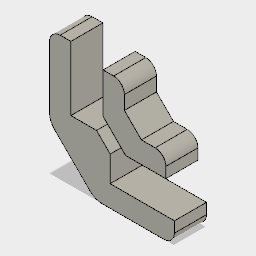
Corner Connector v15 (Autodesk Fusion 360 design; units mm, degrees)
Autodesk Fusion 360 part; units mm, degrees
sketch "Sketch1" plane through (0, 0, 0) normal (0, 0, 1) x (1, 0, 0) in component "InsideClamp"
  line L0 (0, 0) -> (23.8125, 0)
  line L1 (23.8125, 0) -> (37.2829, -13.4704)
  line L2 (37.2829, -13.4704) -> (37.2829, -37.2829)
  line L3 (37.2829, -37.2829) -> (30.9329, -37.2829)
  line L4 (0, 0) -> (0, -6.35)
  line L5 (6.35, -12.7) -> (14.4801, -12.7)
  line L6 (14.4801, -12.7) -> (24.5829, -22.8028)
  line L7 (24.5829, -22.8028) -> (24.5829, -30.9329)
  arc A0 (0, -6.35) -> (6.35, -12.7) centre (6.35, -6.35) ccw
  arc A1 (24.5829, -30.9329) -> (30.9329, -37.2829) centre (30.9329, -30.9329) ccw
  point P0 (24.5829, -37.2829)
  point P1 (0, -12.7)
  dimension "d19" = 23.8125
  dimension "d20" = 19.05
  dimension "d21" = 23.8125
  dimension "d22" = 135
  dimension "d23" = 135
  dimension "d24" = 12.7
  dimension "d25" = 12.7
  dimension "d26" = 135
  dimension "d27" = 135
  dimension "d28" = 14.2875
  dimension "d29" = 6.35
  dimension "d30" = 6.35
  measures "d19" distance of L0.start L0.end
  measures "d20" distance of L0.end L1.end
  measures "d21" distance of L1.end L2.end
  measures "d22" angle of L0 L1
  measures "d23" angle of L1 L2
  measures "d24" distance of L2.end P0
  measures "d25" distance of L0.start P1
  measures "d26" angle of L5 L6
  measures "d27" angle of L6 L7
  measures "d28" distance of L5.end L6.end
  measures "d29" radius of A0
  measures "d30" radius of A1
sketch "Sketch1 (2)" plane through (0, 0, 0) normal (0, 0, 1) x (1, 0, 0) in component "OutsideClamp"
  line L0 (-5.0893, 19.05) -> (33.0107, 19.05)
  line L1 (33.0107, 3.81) -> (41.0929, -4.2722)
  line L2 (56.3329, -4.2722) -> (56.3329, -42.3722)
  line L3 (56.3329, -42.3722) -> (62.6829, -42.3722)
  line L4 (69.0329, -36.0222) -> (69.0329, 0.6008)
  line L5 (66.0571, 7.785) -> (45.0679, 28.7742)
  line L6 (37.8837, 31.75) -> (1.2607, 31.75)
  line L7 (-5.0893, 25.4) -> (-5.0893, 19.05)
  arc A0 (1.2607, 31.75) -> (-5.0893, 25.4) centre (1.2607, 25.4) ccw
  arc A1 (62.6829, -42.3722) -> (69.0329, -36.0222) centre (62.6829, -36.0222) ccw
  line L8 (0, 0) -> (23.8125, 0)
  line L9 (37.2829, -13.4704) -> (37.2829, -37.2829)
  line L10 (33.0107, 19.05) -> (33.0107, 3.81)
  line L11 (56.3329, -4.2722) -> (41.0929, -4.2722)
  arc A2 (45.0679, 28.7742) -> (37.8837, 31.75) centre (37.8837, 21.59) ccw
  arc A3 (69.0329, 0.6008) -> (66.0571, 7.785) centre (58.8729, 0.6008) ccw
  point P0 (69.0329, -42.3722)
  point P1 (69.0329, 4.8092)
  point P2 (42.0921, 31.75)
  point P3 (-5.0893, 31.75)
  dimension "d32" = 38.1
  dimension "d38" = 135
  dimension "d39" = 135
  dimension "d42" = 6.35
  dimension "d43" = 6.35
  dimension "d44" = 12.7
  dimension "d46" = 12.7
  dimension "d47" = 38.1
  dimension "d49" = 19.05
  dimension "d50" = 19.05
  dimension "d51" = 15.24
  dimension "d52" = 15.24
  dimension "d53" = 135
  dimension "d54" = 38.1
  dimension "d55" = 11.43
  dimension "d56" = 10.16
  measures "d32" distance of L0.start L0.end
  measures "d38" angle of L4 L5
  measures "d39" angle of L5 L6
  measures "d42" radius of A0
  measures "d43" radius of A1
  measures "d44" distance of L0 L6
  measures "d46" distance of L2 L4
  measures "d47" distance of P1 P2
  measures "d49" distance of L0 L8
  measures "d50" distance of L2 L9
  measures "d51" distance of L0.end L1.start
  measures "d52" distance of L2.start L1.end
  measures "d53" angle of L1 L10
  measures "d54" distance of L2.end L2.start
  measures "d55" distance of L1.start L1.end
  measures "d56" radius of A2
extrude "Extrude1" add sketch "Sketch1" along normal blind 19.05 makes body 1 in component "InsideClamp"
extrude "Extrude1'" add sketch "Sketch1 (2)" along normal blind 19.05 separate body makes body 2 in component "OutsideClamp"
move_face "MoveFace1" by (0, 5.08, 0) 1 faces at (51.8002, 7.5209, 19.05) on bodies 2 in component "OutsideClamp"
component "InsideClamp" placed x (1, 0, 0) y (0, 1, 0) z (0, 0, 1) at (0, 0, 0)
component "OutsideClamp" placed x (1, 0, 0) y (0, 1, 0) z (0, 0, 1) at (0, 0, 0)
equation "materialThickness = 0.75 in"
equation "d19 = 1.25 * materialThickness"
equation "d20 = materialThickness"
equation "d21 = 1.25 * materialThickness"
equation "d28 = 0.75 * materialThickness"
equation "d32 = 2 * materialThickness"
equation "d47 = 2 * materialThickness"
equation "d49 = materialThickness"
equation "d50 = materialThickness"
equation "d51 = 0.8 * materialThickness"
equation "d52 = 0.8 * materialThickness"
equation "d54 = 2 * materialThickness"
equation "d55 = 0.6 * materialThickness"
equation "d57 = materialThickness"
equation "d59 = materialThickness"
